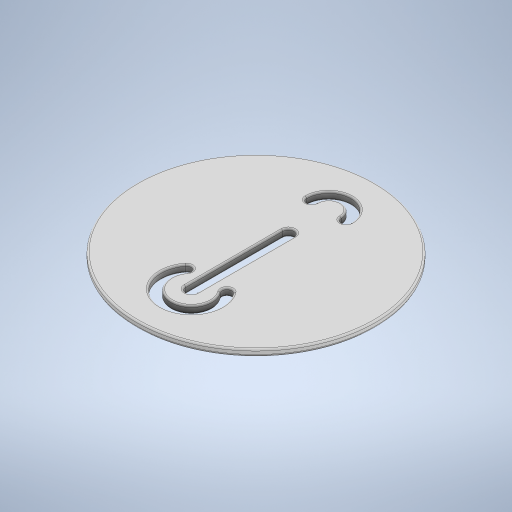
# Autodesk Inventor part: ChamberWireRunSymbolDisc
Saved by Autodesk Inventor 2023 (Build 270158000, 158)
## iProperties
Created: 2026-02-18
Part Number: ChamberWireRunSymbolDisc
Material: Generic
Document SubType Name: Modeling
Designer: DanAr
Density: 1 g/cm^3
Appearance: Default
Author: DanAr
Autodesk Inventor part; units mm, degrees
ref_plane "YZ Plane" through (0, 0, 0) normal (1, 0, 0) x (0, 1, 0)
ref_plane "XZ Plane" through (0, 0, 0) normal (0, 1, 0) x (-1, 0, 0)
ref_plane "XY Plane" through (0, 0, 0) normal (0, 0, 1) x (1, 0, 0)
sketch "Sketch1" plane through (0, 0, 0) normal (0, 1, 0) x (-1, 0, 0)
  circle A0 centre (0, 0.7751) radius 14.8
  line L0 (0, 0.7751) -> (0, 2.7751)
  line L1 (0, 8.7751) -> (0, -3.2249) construction
  line L2 (-0.7, 8.7751) -> (-0.7, -3.2249)
  line L3 (0.7, -3.2249) -> (0.7, 8.7751)
  arc A1 (0.7, 8.7751) -> (-0.7, 8.7751) centre (0, 8.7751) ccw
  arc A2 (-0.7, -3.2249) -> (0.7, -3.2249) centre (0, -3.2249) ccw
  circle A3 centre (0, 8.7751) radius 3.141
  line L4 (0, 8.7751) -> (-2.5128, 6.8905)
  line L5 (0, 8.7751) -> (2.5128, 6.8905)
  arc A4 (2.5128, 6.8905) -> (-2.5128, 6.8905) centre (0, 8.7751) ccw construction
  arc A5 (2.9928, 6.5305) -> (-2.9928, 6.5305) centre (0, 8.7751) ccw
  arc A6 (2.0328, 7.2505) -> (-2.0328, 7.2505) centre (0, 8.7751) ccw
  arc A7 (2.0328, 7.2505) -> (2.9928, 6.5305) centre (2.5128, 6.8905) ccw
  arc A8 (-2.9928, 6.5305) -> (-2.0328, 7.2505) centre (-2.5128, 6.8905) ccw
  line L6 (0, 0.7751) -> (-2.141, 0.7751)
  line L7 (-2.141, 0.7751) -> (-2.141, -8.2249)
  line L8 (-2.141, -8.2249) -> (0, -8.2249)
  line L9 (0, -8.2249) -> (0, 0.7751)
  arc A9 (-2.141, -8.2249) -> (2.141, -8.2249) centre (0, -8.2249) ccw construction
  arc A10 (-2.741, -8.2249) -> (2.741, -8.2249) centre (0, -8.2249) ccw
  arc A11 (-1.541, -8.2249) -> (1.541, -8.2249) centre (0, -8.2249) ccw
  arc A12 (-1.541, -8.2249) -> (-2.741, -8.2249) centre (-2.141, -8.2249) ccw
  arc A13 (2.741, -8.2249) -> (1.541, -8.2249) centre (2.141, -8.2249) ccw
  dimension "d0" = 29.6
  dimension "d2" = 2
  dimension "d3" = 0.7
  dimension "d4" = 12
  dimension "d5" = 6.282
  dimension "d6" = 53.13
  dimension "d7" = 106.26
  dimension "d8" = 0.6
  dimension "d9" = 9
  dimension "d10" = 2.141
  dimension "d11" = 0.6
  constraints: 26 point on circle, 22 end point, 14 centre point, 12 tangent, 3 coincident, 3 parallel, 2 vertical, 1 horizontal, 1 midpoint, 1 perpendicular
  measures "d0" diameter of A0
  measures "d2" distance of L0.start L0.end
  measures "d3" radius of A2
  measures "d4" distance of L1.start L1.end
  measures "d5" diameter of A3
  measures "d6" angle of L1 L4
  measures "d7" angle of L4 L5
  measures "d8" radius of A7
  measures "d9" distance of L6.end L7.end
  measures "d10" distance of L7.end L8.end
  measures "d11" radius of A13
extrude "Extrusion1" add sketch "Sketch1" along normal blind 0.95 contours A0 | L2 L4 A6 L5 L3 A1 | L2 A3 A8 L4 | L5 A7 A3 L3 | L2 A2 L9 L8 A12 L7 L6
chamfer "Chamfer1" distance 0.3 angle 45 1 edges at (14.8, 0, 0.7751)
fillet "Fillet1" radius 0.2 27 edges at (14.8, 0.95, 0.7751) (-2.1528, 0.95, 6.4105) (0, 0.95, 11.3161) (2.1528, 0.95, 6.4105) (0, 0.95, 12.5161) (0, 0.95, -3.9249) (0.7, 0.95, 2.7751) (0, 0.95, 9.4751) (-0.7, 0.95, 2.7751) (-2.141, 0.95, -7.6249) (0, 0.95, -10.9659) (2.141, 0.95, -7.6249) (0, 0.95, -9.7659) (0, 0, 12.5161) (-2.1528, 0, 6.4105) (0, 0, 11.3161) (2.1528, 0, 6.4105) (0, 0, 9.4751) (-0.7, 0, 2.7751) (0, 0, -3.9249) (0.7, 0, 2.7751) (2.141, 0, -7.6249) (0, 0, -9.7659) (-2.141, 0, -7.6249) (0, 0, -10.9659) (14.8, 0.3, 0.7751) (14.5, 0, 0.7751)
body "Solid1"
